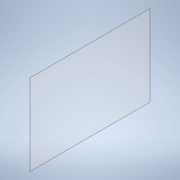
# Autodesk Inventor part: StationWindow-ver1-1111-2021
Saved by Autodesk Inventor 2021 (Build 250183000, 183)
## iProperties
Created: 2021-03-02
Part Number: StationWindow-ver1-1111-2021
Material: Generic
Document SubType Name: Modeling
Designer: CMurray
Density: 1 g/cm^3
Appearance: Polycarbonate - Clear
Author: CMurray
Autodesk Inventor part; units mm, degrees
ref_plane "YZ Plane" through (0, 0, 0) normal (1, 0, 0) x (0, 1, 0)
ref_plane "XZ Plane" through (0, 0, 0) normal (0, 1, 0) x (-1, 0, 0)
ref_plane "XY Plane" through (0, 0, 0) normal (0, 0, 1) x (1, 0, 0)
sketch "Sketch1" plane through (0, 0, 0) normal (1, 0, 0) x (0, 1, 0)
  line L0 (0, 0) -> (1028.7, 0)
  line L1 (1028.7, 0) -> (1028.7, -1524)
  line L2 (1028.7, -1524) -> (0, -1524)
  line L3 (0, -1524) -> (0, 0)
  dimension "d2" = 1524
  dimension "d3" = 1028.7
  constraints: 8 end point, 2 parallel, 1 horizontal, 1 perpendicular
  measures "d2" distance between parallel lines of L2 L0
  measures "d3" distance between parallel lines of L3 L1
extrude "Extrusion1" add sketch "Sketch1" along normal blind 3.175
body "Solid1"
